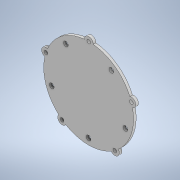
# Autodesk Inventor part: Base_Suelo
Saved by Autodesk Inventor 2022 (Build 260153000, 153)
## iProperties
Created: 2021-09-09
Part Number: Base_Suelo
Material: Generic
Document SubType Name: Modeling
Designer: Administrador
Density: 1 g/cm^3
Appearance: Default
Author: Administrador
Autodesk Inventor part; units mm, degrees
ref_plane "YZ Plane" through (0, 0, 0) normal (1, 0, 0) x (0, 1, 0)
ref_plane "XZ Plane" through (0, 0, 0) normal (0, 1, 0) x (-1, 0, 0)
ref_plane "XY Plane" through (0, 0, 0) normal (0, 0, 1) x (1, 0, 0)
sketch "Sketch1" plane through (0, 0, 0) normal (0, 1, 0) x (-1, 0, 0)
  point P0 (0, 0)
sketch "Sketch2" plane through (0, 0, 0) normal (0, 0, 1) x (1, 0, 0)
  circle A0 centre (0, -44) radius 2.7
  circle A1 centre (-41.8465, -13.5967) radius 2.7
  circle A2 centre (-25.8626, 35.5967) radius 2.7
  circle A3 centre (25.8626, 35.5967) radius 2.7
  circle A4 centre (41.8465, -13.5967) radius 2.7
  arc A5 (5.1973, 50.7345) -> (-4.7916, 50.7744) centre (0.2038, 50.9896) ccw
  circle A6 centre (0.2038, 50.9896) radius 2.1
  arc A7 (0.2038, 50.9896) -> (-1.8959, 50.9547) centre (0, 0) ccw
  arc A8 (-2.6987, -43.9172) -> (0, -44) centre (0, 0) ccw
  arc A9 (-46.6453, 20.6207) -> (-49.77, 11.1331) centre (-48.431, 15.9505) ccw
  circle A10 centre (-48.431, 15.9505) radius 2.1
  arc A11 (-34.0257, -37.9902) -> (-25.968, -43.8938) centre (-30.1358, -41.1316) ccw
  circle A12 centre (-30.1358, -41.1316) radius 2.1
  arc A13 (25.6163, -44.1) -> (33.7209, -38.261) centre (29.806, -41.3712) ccw
  circle A14 centre (29.806, -41.3712) radius 2.1
  arc A15 (49.8574, 10.7349) -> (46.8087, 20.2472) centre (48.557, 15.5628) ccw
  circle A16 centre (48.557, 15.5628) radius 2.1
  arc A17 (-4.7916, 50.7744) -> (-46.6453, 20.6207) centre (0, 0) ccw
  arc A18 (-49.77, 11.1331) -> (-34.0257, -37.9902) centre (0, 0) ccw
  arc A19 (-25.968, -43.8938) -> (25.6163, -44.1) centre (0, 0) ccw
  arc A20 (33.7209, -38.261) -> (49.8574, 10.7349) centre (0, 0) ccw
  arc A21 (46.8087, 20.2472) -> (5.1973, 50.7345) centre (0, 0) ccw
  point P0 (2.3032, 50.9382)
  point P1 (-49.0467, 13.9428)
  point P2 (-47.7333, 17.9312)
  point P3 (-31.804, -39.8561)
  point P4 (28.0774, -42.5636)
  point P5 (49.1568, 13.5503)
  point P6 (-28.4166, -42.3376)
  point P7 (31.4843, -40.1089)
  point P8 (47.875, 17.549)
  dimension "d2" = 5.4
  dimension "d5" = 360
  dimension "d7" = 10
  dimension "d8" = 4.2
  dimension "d11" = 360
  dimension "d15" = 51
  constraints: 34 point on circle, 21 centre point, 8 coincident, 55 other
  measures "d7" diameter of A5
  measures "d8" diameter of A6
  measures "d15" radius of A17
extrude "BaseSuelo" add sketch "Sketch2" along normal blind 3
body "Solid1"
